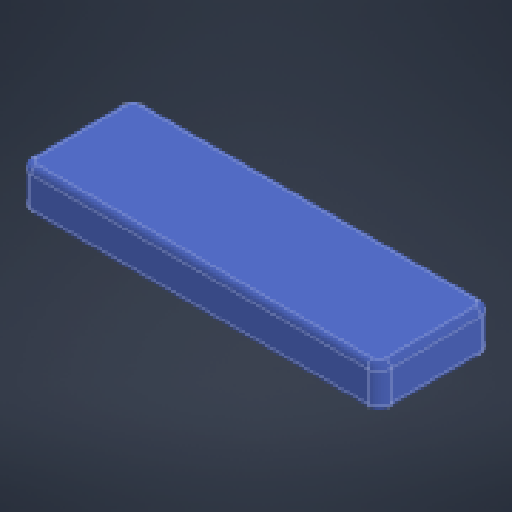
# Autodesk Inventor part: P_Akku_1S
Saved by Autodesk Inventor 2026 (Build 300175000, 175)
## iProperties
Created: 2025-08-01
Part Number: P_Akku_1S
Material: Generisch
Document SubType Name: Modeling
Designer: FAL
Density: 1 g/cm^3
Appearance: Vorgabe
Author: FAL
Autodesk Inventor part; units mm, degrees
ref_plane "YZ Plane" through (0, 0, 0) normal (1, 0, 0) x (0, 1, 0)
ref_plane "XZ Plane" through (0, 0, 0) normal (0, 1, 0) x (-1, 0, 0)
ref_plane "XY Plane" through (0, 0, 0) normal (0, 0, 1) x (1, 0, 0)
sketch "Skizze1" plane through (0, 0, 0) normal (0, 0, 1) x (1, 0, 0)
  line L0 (30, 9.5) -> (-30, 9.5)
  line L1 (-30, 9.5) -> (-30, -9.5)
  line L2 (-30, -9.5) -> (30, -9.5)
  line L3 (30, -9.5) -> (30, 9.5)
  line L4 (30, 9.5) -> (-30, -9.5) construction
  line L5 (-30, 9.5) -> (30, -9.5) construction
  point P0 (0, 0)
  dimension "d0" = 60
  dimension "d1" = 19
  constraints: 12 end point, 2 midpoint, 2 parallel, 1 horizontal, 1 perpendicular
  measures "d0" distance of L0.start L0.end
  measures "d1" distance of L0.end L1.end
extrude "Extrusion1" add sketch "Skizze1" along normal blind 7
fillet "Rundung1" radius 2 4 edges at (-30, -9.5, 3.5) (30, -9.5, 3.5) (30, 9.5, 3.5) (-30, 9.5, 3.5)
fillet "Rundung2" radius 1 16 edges at (-29.4142, 8.9142, 7) (-30, 0, 7) (-29.4142, -8.9142, 7) (0, -9.5, 7) (29.4142, -8.9142, 7) (30, 0, 7) (29.4142, 8.9142, 7) (0, 9.5, 7) (29.4142, -8.9142, 0) (30, 0, 0) (29.4142, 8.9142, 0) (0, 9.5, 0) (-29.4142, 8.9142, 0) (-30, 0, 0) (-29.4142, -8.9142, 0) (0, -9.5, 0)
